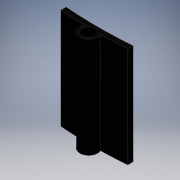
# Autodesk Inventor part: ET24
Saved by Autodesk Inventor 2016 (Build 200138000, 138)
## iProperties
Created: 2016-04-18
Part Number: ET24
Material: Genérico
Document SubType Name: Modeling
Designer: Usuario1
Density: 1 g/cm^3
Appearance: Valor por defecto
Author: Usuario1
Autodesk Inventor part; units mm, degrees
ref_plane "YZ Plane" through (0, 0, 0) normal (1, 0, 0) x (0, 1, 0)
ref_plane "XZ Plane" through (0, 0, 0) normal (0, 1, 0) x (-1, 0, 0)
ref_plane "XY Plane" through (0, 0, 0) normal (0, 0, 1) x (1, 0, 0)
sketch "Boceto1" plane through (0, 0, 0) normal (0, 0, 1) x (1, 0, 0)
  arc A0 (0.7874, 0.8092) -> (2.7771, 0.8092) centre (1.7822, 6.8708) ccw
  circle A1 centre (1.774, 0.5957) radius 0.0981
  circle A2 centre (1.774, 0.5957) radius 0.1324
  line L0 (2.2809, 0.7484) -> (2.2809, 0.67)
  line L1 (1.2836, 0.7484) -> (1.2836, 0.67)
  arc A3 (1.2836, 0.67) -> (1.6537, 0.651) centre (1.7822, 6.7924) ccw
  arc A4 (1.8945, 0.6507) -> (2.2809, 0.67) centre (1.7822, 6.7924) ccw
  point P0 (0, 0)
  constraints: 10 point on circle, 5 centre point, 4 end point
extrude "Extrusión1" add sketch "Boceto1" along normal blind 1.5
